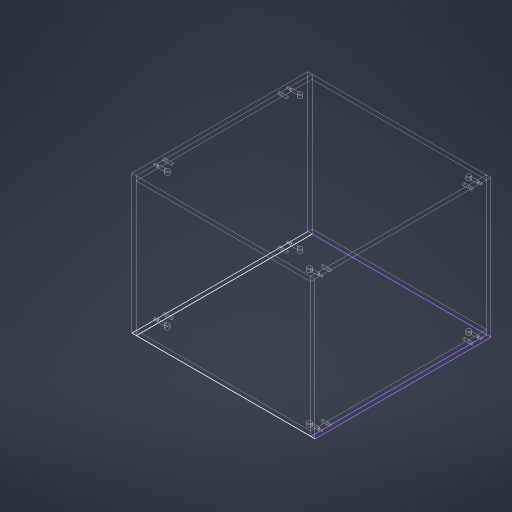
# Autodesk Inventor part: Деталь1
Saved by Autodesk Inventor 2023.4 (Build 274418000, 418)
## iProperties
Created: 2026-09-26
Part Number: Деталь1
Material: Типовые
Document SubType Name: Modeling
Designer: desig
Density: 1 g/cm^3
Appearance: По умолчанию
Author: desig
Autodesk Inventor part; units mm, degrees
ref_plane "YZ Plane" through (0, 0, 0) normal (1, 0, 0) x (0, 1, 0)
ref_plane "XZ Plane" through (0, 0, 0) normal (0, 1, 0) x (-1, 0, 0)
ref_plane "XY Plane" through (0, 0, 0) normal (0, 0, 1) x (1, 0, 0)
sketch "Эскиз1" plane through (0, 0, 0) normal (0, 1, 0) x (-1, 0, 0)
  line L0 (0, 0) -> (-16, 0)
  line L1 (-16, 0) -> (-16, -636.0264)
  line L2 (-16, -636.0264) -> (0, -636.0264)
  line L3 (0, -636.0264) -> (0, 0)
  line L4 (-646.4743, 0) -> (-662.4743, 0)
  line L5 (-662.4743, 0) -> (-662.4743, -636.0264)
  line L6 (-662.4743, -636.0264) -> (-646.4743, -636.0264)
  line L7 (-646.4743, -636.0264) -> (-646.4743, 0)
  line L8 (-16, -636.0264) -> (-646.4743, -636.0264)
  line L9 (-16, 0) -> (-646.4743, 0)
  dimension "d0" = 16
  dimension "d1" = 16
  dimension "d46" = 636.026
  dimension "d47" = 662.474
  constraints: 20 end point, 4 parallel, 3 horizontal, 3 perpendicular, 2 point on line
  measures "d0" distance of L1.end L2.end
  measures "d1" distance of L5.end L6.end
  measures "d46" distance of L2.end L0.start
  measures "d47" distance between parallel lines of L5 L3
extrude "Выдавливание1" add sketch "Эскиз1" along normal blind 500 contours L3 L2 L1 L0
extrude "Выдавливание2" add sketch "Эскиз1" against normal blind 16 from surface at 500 separate body contours L1 L8 L7 L9
extrude "Выдавливание3" add sketch "Эскиз1" along normal blind 16 separate body contours L1 L8 L7 L9
extrude "Выдавливание4" add sketch "Эскиз1" along normal up to surface (500 mm away) separate body contours L7 L6 L5 L4
sketch "DrillingSketch_1" plane through (16, 484, 0) normal (-1, 0, 0) x (0, 0, 1)
  line L0 (0, 0) -> (-636.0264, 0) projected
  line L1 (0, 16) -> (0, 0) projected
  line L2 (0, 16) -> (-636.0264, 16) projected
  line L3 (-636.0264, 0) -> (-636.0264, 16) projected
  line L4 (0, 8) -> (-636.0264, 8) construction
  line L5 (-318.0132, 8) -> (-318.0132, -12) construction
  line L6 (-636.0264, -484) -> (0, -484) projected
  line L7 (0, -484) -> (0, -468) projected
  line L8 (-636.0264, -468) -> (0, -468) projected
  line L9 (-636.0264, -484) -> (-636.0264, -468) projected
  line L10 (0, -476) -> (-636.0264, -476) construction
  line L11 (-318.0132, -476) -> (-318.0132, -496) construction
  point P0 (-78.0132, 8)
  point P1 (-558.0132, 8)
  point P2 (-110.0132, 8)
  point P3 (-526.0132, 8)
  point P4 (-78.0132, -476)
  point P5 (-558.0132, -476)
  point P6 (-110.0132, -476)
  point P7 (-526.0132, -476)
  dimension "Минимальный_отступ_присадки_от_кромки_Каркас" = 70
  dimension "Long_edge_1" = 636.0264
  dimension "Расстояние_между_точками" = 480
  dimension "d2004" = 32
  dimension "Long_edge_2" = 636.0264
  dimension "Расстояние_между_точками_2" = 480
  dimension "d2007" = 32
  constraints: 10 point on line, 8 end point, 8 midpoint, 4 symmetric about line, 2 perpendicular
  measures "Long_edge_1" distance of L4.start L4.end
  measures "Расстояние_между_точками" distance of point (-558.013, 8) point (-78.013, 8)
  measures "d2004" distance of point (-78.013, 8) point (-110.013, 8)
  measures "Long_edge_2" distance of L10.start L10.end
  measures "Расстояние_между_точками_2" distance of point (-558.013, -476) point (-78.013, -476)
  measures "d2007" distance of point (-78.013, -476) point (-110.013, -476)
sketch "DrawerSketch_1" plane through (646.4743, 484, -636.0264) normal (1, 0, 0) x (0, 0, -1)
  line L0 (0, 0) -> (-636.0264, 0) projected
  line L1 (0, 0) -> (0, 16) projected
  line L2 (0, 16) -> (-636.0264, 16) projected
  line L3 (-636.0264, 0) -> (-636.0264, 16) projected
  line L4 (0, 8) -> (-636.0264, 8) construction
  line L5 (-318.0132, 8) -> (-318.0132, -12) construction
  line L6 (-636.0264, -484) -> (0, -484) projected
  line L7 (0, -484) -> (0, -468) projected
  line L8 (-636.0264, -468) -> (0, -468) projected
  line L9 (-636.0264, -484) -> (-636.0264, -468) projected
  line L10 (0, -476) -> (-636.0264, -476) construction
  line L11 (-318.0132, -476) -> (-318.0132, -496) construction
  point P0 (-30.0132, 8)
  point P1 (-606.0132, 8)
  point P2 (-62.0132, 8)
  point P3 (-574.0132, 8)
  point P4 (-30.0132, -476)
  point P5 (-606.0132, -476)
  point P6 (-62.0132, -476)
  point P7 (-574.0132, -476)
  dimension "d46" = 636.026
  dimension "d47" = 662.474
  dimension "Минимальный_отступ_присадки_от_кромки_Ящик" = 20
  dimension "Long_edge_1_2" = 636.0264
  dimension "Расстояние_между_точками_3" = 576
  dimension "d2010" = 32
  dimension "Long_edge_2_2" = 636.0264
  dimension "Расстояние_между_точками_4" = 576
  dimension "d2013" = 32
  constraints: 10 point on line, 8 end point, 8 midpoint, 4 symmetric about line, 2 perpendicular
  measures "Long_edge_1_2" distance of L4.start L4.end
  measures "Расстояние_между_точками_3" distance of point (-606.013, 8) point (-30.013, 8)
  measures "d2010" distance of point (-30.013, 8) point (-62.013, 8)
  measures "Long_edge_2_2" distance of L10.start L10.end
  measures "Расстояние_между_точками_4" distance of point (-606.013, -476) point (-30.013, -476)
  measures "d2013" distance of point (-30.013, -476) point (-62.013, -476)
hole "Stiajka outer 8x34" at (16, 492, -78.0132) at (16, 492, -558.0132) direction (1, 0, 0) diameter 8 depth 34 bodies 1 2 3 4
hole "Stiajka outer 5x13" at (16, 492, -78.0132) at (16, 492, -558.0132) direction (-1, 0, 0) diameter 5 depth 12.5 bodies 1 2 3 4
hole "Shkant 8x10" at (16, 492, -110.0132) at (16, 492, -526.0132) direction (-1, 0, 0) diameter 8 depth 10 bodies 1 2 3 4
hole "Shkant 8x20" at (16, 492, -110.0132) at (16, 492, -526.0132) direction (1, 0, 0) diameter 8 depth 20 bodies 1 2 3 4
sketch "StiajkaSideSketch" plane through (16, 484, 0) normal (0, -1, 0) x (1, 0, 0)
  line L0 (0, -82.0132) -> (0, -74.0132) projected
  line L1 (34, -74.0132) -> (34, -82.0132) projected
  line L2 (0, -562.0132) -> (0, -554.0132) projected
  line L3 (34, -554.0132) -> (34, -562.0132) projected
  point P0 (34, -78.0132)
  point P1 (34, -558.0132)
  dimension "d46" = 636.026
  dimension "d47" = 662.474
  constraints: 2 midpoint
hole "Stiajka cup" at (50, 484, -78.0132) at (50, 484, -558.0132) direction (0, 1, 0) diameter 15 depth 12.5 bodies 1 2 3 4
hole "Stiajka outer 8x34 2" at (16, 8, -78.0132) at (16, 8, -558.0132) direction (1, 0, 0) diameter 8 depth 34 bodies 1 2 3 4
hole "Stiajka outer 5x13 2" at (16, 8, -78.0132) at (16, 8, -558.0132) direction (-1, 0, 0) diameter 5 depth 12.5 bodies 1 2 3 4
hole "Shkant 8x10 2" at (16, 8, -110.0132) at (16, 8, -526.0132) direction (-1, 0, 0) diameter 8 depth 10 bodies 1 2 3 4
hole "Shkant 8x20 2" at (16, 8, -110.0132) at (16, 8, -526.0132) direction (1, 0, 0) diameter 8 depth 20 bodies 1 2 3 4
sketch "StiajkaSideSketch_2" plane through (0, 0, 0) normal (0, -1, 0) x (1, 0, 0)
  line L0 (16, -82.0132) -> (16, -74.0132) projected
  line L1 (50, -74.0132) -> (50, -82.0132) projected
  line L2 (16, -562.0132) -> (16, -554.0132) projected
  line L3 (50, -554.0132) -> (50, -562.0132) projected
  point P0 (50, -78.0132)
  point P1 (50, -558.0132)
  dimension "d46" = 636.026
  dimension "d47" = 662.474
  constraints: 2 midpoint
hole "Stiajka cup 2" at (50, 0, -78.0132) at (50, 0, -558.0132) direction (0, 1, 0) diameter 15 depth 12.5 bodies 1 2 3 4
hole "Stiajka outer 8x34 3" at (646.4743, 492, -606.0132) at (646.4743, 492, -30.0132) direction (-1, 0, 0) diameter 8 depth 34 bodies 1 2 3 4
hole "Stiajka outer 5x13 3" at (646.4743, 492, -606.0132) at (646.4743, 492, -30.0132) direction (1, 0, 0) diameter 5 depth 12.5 bodies 1 2 3 4
hole "Shkant 8x10 3" at (646.4743, 492, -574.0132) at (646.4743, 492, -62.0132) direction (1, 0, 0) diameter 8 depth 10 bodies 1 2 3 4
hole "Shkant 8x20 3" at (646.4743, 492, -574.0132) at (646.4743, 492, -62.0132) direction (-1, 0, 0) diameter 8 depth 20 bodies 1 2 3 4
sketch "StiajkaSideSketch_3" plane through (16, 484, 0) normal (0, -1, 0) x (1, 0, 0)
  line L0 (630.4743, -602.0132) -> (630.4743, -610.0132) projected
  line L1 (596.4743, -610.0132) -> (596.4743, -602.0132) projected
  line L2 (630.4743, -26.0132) -> (630.4743, -34.0132) projected
  line L3 (596.4743, -34.0132) -> (596.4743, -26.0132) projected
  point P0 (596.4743, -606.0132)
  point P1 (596.4743, -30.0132)
  dimension "d46" = 636.026
  dimension "d47" = 662.474
  constraints: 2 midpoint
hole "Stiajka cup 3" at (612.4743, 484, -606.0132) at (612.4743, 484, -30.0132) direction (0, 1, 0) diameter 15 depth 12.5 bodies 1 2 3 4
hole "Stiajka outer 8x34 4" at (646.4743, 8, -606.0132) at (646.4743, 8, -30.0132) direction (-1, 0, 0) diameter 8 depth 34 bodies 1 2 3 4
hole "Stiajka outer 5x13 4" at (646.4743, 8, -606.0132) at (646.4743, 8, -30.0132) direction (1, 0, 0) diameter 5 depth 12.5 bodies 1 2 3 4
hole "Shkant 8x10 4" at (646.4743, 8, -574.0132) at (646.4743, 8, -62.0132) direction (1, 0, 0) diameter 8 depth 10 bodies 1 2 3 4
hole "Shkant 8x20 4" at (646.4743, 8, -574.0132) at (646.4743, 8, -62.0132) direction (-1, 0, 0) diameter 8 depth 20 bodies 1 2 3 4
sketch "StiajkaSideSketch_4" plane through (0, 0, 0) normal (0, -1, 0) x (1, 0, 0)
  line L0 (646.4743, -602.0132) -> (646.4743, -610.0132) projected
  line L1 (612.4743, -610.0132) -> (612.4743, -602.0132) projected
  line L2 (646.4743, -26.0132) -> (646.4743, -34.0132) projected
  line L3 (612.4743, -34.0132) -> (612.4743, -26.0132) projected
  point P0 (612.4743, -606.0132)
  point P1 (612.4743, -30.0132)
  dimension "d46" = 636.026
  dimension "d47" = 662.474
  constraints: 2 midpoint
hole "Stiajka cup 4" at (612.4743, 0, -606.0132) at (612.4743, 0, -30.0132) direction (0, 1, 0) diameter 15 depth 12.5 bodies 1 2 3 4
equation "\"d0\" = Толщина_каркаса"
equation "\"d1\" = Толщина_каркаса"
equation "\"d5\" = Толщина_каркаса"
equation "\"d7\" = Толщина_каркаса"
equation "\"Минимальный_отступ_присадки_от_кромки_Каркас\" = 70"
equation "\"Минимальный_отступ_присадки_от_кромки_Ящик\" = 20"
equation "\"Толщина_каркаса\" = 16"
equation "\"Стяжка_D\" = 15"
equation "\"Стяжка_h\" = 12.5"
equation "\"Стяжка_D_резьбыШтока\" = 5"
equation "\"Стяжка_D_телаШтока\" = 8"
equation "\"Стяжка_резьбыШтока_Петля_h\" = 12.5"
equation "\"Стяжка_отступ\" = 34"
equation "\"Конфирмат_D_вПласть\" = 8"
equation "\"Конфирмат_D_вТорец\" = 5"
equation "\"Толщина_каркаса_ящика\" = 16"
equation "\"Шкант_D\" = 8"
equation "\"Полкодержатель_D\" = 5"
equation "\"Полкодержатель_смещение_от_низа_полки\" = 5"
equation "\"Петля_D_присадки\" = 35"
equation "\"M_Конфирмат_глубина_резьбы\" = 35"
equation "\"M_Конфирмат_D_вПласть\" = 5"
equation "\"M_Конфирмат_D_вТорец\" = 3"
equation "\"Толщина_задн_ст_Володя\" = 3"
equation "\"Толщина_дна_ящика_Володя\" = 6"
equation "\"Минимальное_расстояния_от_заднСт_ящика_до_заднСт\" = 25"
equation "\"Западание_кромки_полки_за_каркас\" = 5"
